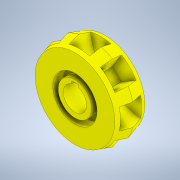
# Autodesk Inventor part: omniwheel
Saved by Autodesk Inventor 2020.2 (Build 242310000, 310)
## iProperties
Created: 2020-03-22
Part Number: omniwheel
Material: Generic
Document SubType Name: Modeling
Designer: Tarsoly
Density: 1 g/cm^3
Appearance: Default
Author: Tarsoly
Autodesk Inventor part; units mm, degrees
ref_plane "YZ Plane" through (0, 0, 0) normal (1, 0, 0) x (0, 1, 0)
ref_plane "XZ Plane" through (0, 0, 0) normal (0, 1, 0) x (-1, 0, 0)
ref_plane "XY Plane" through (0, 0, 0) normal (0, 0, 1) x (1, 0, 0)
sketch "Sketch1" plane through (0, 0, 0) normal (0, 0, 1) x (1, 0, 0)
  circle A0 centre (0, 0) radius 22.5
  dimension "d0" = 45
  constraints: 1 centre point, 1 coincident
  measures "d0" diameter of A0
extrude "Extrusion1" add sketch "Sketch1" along normal mid plane 17
sketch "Sketch2" plane through (0, 0, 8.5) normal (0, 0, 1) x (1, 0, 0)
  circle A0 centre (0, 0) radius 6.6
  line L0 (-1.75, 7.8638) -> (1.75, 7.8638)
  line L1 (1.75, 7.8638) -> (1.75, 6.3638)
  line L2 (1.75, 6.3638) -> (-1.75, 6.3638)
  line L3 (-1.75, 6.3638) -> (-1.75, 7.8638)
  dimension "d3" = 13.2
  dimension "d4" = 3.5
  dimension "d5" = 1.5
  constraints: 8 end point, 2 parallel, 2 point on circle, 1 centre point, 1 coincident, 1 horizontal, 1 perpendicular
  measures "d3" diameter of A0
  measures "d4" distance of L1.end L2.end
  measures "d5" distance of L0.end L1.end
extrude "Extrusion2" cut sketch "Sketch2" against normal through all
sketch "Sketch3" plane through (0, 0, 8.5) normal (0, 0, 1) x (1, 0, 0)
  circle A0 centre (0, 0) radius 9.5
  circle A1 centre (0, 0) radius 12.5
  dimension "d8" = 19
  dimension "d9" = 3
  constraints: 2 centre point, 1 coincident
  measures "d8" diameter of A0
  measures "d9" radial gap between concentric circles of A0 A1
extrude "Extrusion3" cut sketch "Sketch3" against normal blind 6
mirror "Mirror1" about plane through (0, 0, 0) normal (0, 0, 1) of "Extrusion3"
sketch "Sketch4" plane through (0, 0, 0) normal (0, 1, 0) x (-1, 0, 0)
  line L0 (22.5, -8.5) -> (22.5, 8.5) projected
  line L1 (22.5, -8.5) -> (25, 0)
  line L2 (25, 0) -> (22.5, 8.5)
  line L3 (-22.5, -8.5) -> (22.5, -8.5) projected
  line L4 (34.5, 0) -> (-32, 0) projected
  line L5 (0, -11.9) -> (0, 11.9) projected
  point P0 (0, 0)
  dimension "d12" = 2.5
  constraints: 5 point on line, 4 end point
  measures "d12" distance from line of L0 L1.end
revolve "Revolution1" add sketch "Sketch4" angle 360 about axis through (0, 0, -10) along (0, 0, 1) contours L0 L4 L1 | L0 L2 L4
sketch "Sketch5" plane through (0, 0, 0) normal (0, 0, 1) x (1, 0, 0)
  line L0 (-6.5, 25) -> (-3.38, 13)
  line L1 (-3.38, 13) -> (3.38, 13)
  line L2 (3.38, 13) -> (6.5, 25)
  line L3 (6.5, 25) -> (-6.5, 25)
  circle A0 centre (0, 0) radius 25 construction
  line L4 (0, -35) -> (0, 35) construction
  point P0 (0, 13)
  point P1 (0, 25)
  dimension "d14" = 13
  dimension "d15" = 12
  constraints: 8 end point, 2 horizontal, 2 line through centre, 2 midpoint, 2 point on line, 1 tangent
  measures "d14" distance of L2.end L0.start
  measures "d15" distance between parallel lines of L1 L3
extrude "Extrusion4" cut sketch "Sketch5" along normal mid plane 12
pattern_circular "Circular Pattern1" count 8 over 360 about axis through (0, 0, -10) along (0, 0, 1) of "Extrusion4"
sketch "Sketch6" plane through (0, 0, 0) normal (0, 0, 1) x (1, 0, 0)
  circle A0 centre (0, 0) radius 20.5
  dimension "d21" = 41
  constraints: 1 centre point, 1 coincident
  measures "d21" diameter of A0
body "Solid1"
